Autodesk Fusion 360 part; units mm, degrees
(part 2 of 2)
  constraint equal A46 A113
  constraint equal A46 A102
  constraint equal A46 A91
  constraint equal A46 A108
  constraint equal A46 A95
  constraint equal A46 A130
  constraint equal A142 A148
  constraint equal A148 A166
  constraint equal A148 A164
  constraint equal A148 A174
  constraint equal A148 A172
  constraint equal A148 A158
  constraint equal A148 A156
  constraint coincident L101 L185.end
  measures "d19" distance of L0.end L6.end
  measures "d20" distance of L8.end L11.end
  measures "d51" distance of L0.end L8.end
  measures "d144" distance of L78.start L78.end
  measures "d168" distance of L114.end L115.end
  measures "d179" distance of L159.start L159.end
  measures "d275" diameter of A69
  measures "d276" diameter of A149
  measures "d277" diameter of A179
  measures "d279" diameter of A246
  measures "d280" diameter of A185
  measures "d281" diameter of A187
  measures "d282" diameter of A46
  measures "d283" diameter of A148
extrude "Extrude4" cut sketch "Sketch2" against normal blind 3 contours A46 | A53 | A57 | A58 | A59 | A62 | A63 | A64 | A67 | A68 | A69 | A72 | A73 | A74 | A76 | A77 | A78 | A82 | A83 | A84 | A89 | A91 | A93 | A95 | A97 A120 A139 | A99 | A102 | A104 | A105 | A108 | A111 | A112 | A113 | A116 | A117 | A121 | A124 | A125 | A126 | A129 | A130 | A131 | A134 | A135 | A136 | A141 | A142 | A145 | A147 | A148 | A149 | A155 | A156 | A157 | A158 | A159 | A163 | A164 | A165 | A166 | A167 | A171 | A172 | A173 | A174 | A175 | A201 | A202 | A206 | A207 | A208 | A209 | A210 | A214 | A215 | A216 | A217 | A218 | A219 | A220 | A224 | A225 | A226 | A227 | A228 | A229 | A230 | A234 | A235 | A236 | A237 | A238 | A239 | A240 | A241 | A242 | A243 | A244 | A245 | A246 | A253 | A254 | A255 | A258 | A259 | A260 | A263 | A264 | A265 | A268 | A269 | A270 | A273 | A274 | A275 | A280 | A281 bodies 1
extrude "Extrude5" add sketch "Sketch2" along normal blind 3 separate body contours L0 L5 L34 L35 L36 L37 L107 | L0 L35 L81 L104 L105 L106 L107 | L5 L12 L13 L51 L81 L107 L109 L227 | L0 L7 L81 L100 L101 L102 L103 | L0 L1 L6 L7 L8 L9 L103 | L12 L79 L81 L106 A262 A271 | L10 L79 L81 L102 A261 A267 | L81 L223 A261 L224 A262 | L12 L79 L80 L94 A272 | L1 L10 L11 L48 L81 L103 L108 L226 | L79 L223 A262 | L12 A271 L227 A272 L228 | L79 A272 L228 | L79 L93 L94 L95 A257 | L86 A123 L153 L156 L157 L158 | L10 L225 A266 A267 L226 | L79 L225 A267 | L95 L221 A257 | L93 L221 A256 L222 A257 | L86 A127 L152 L153 | L10 L78 L79 L90 A266 | A75 L93 L95 A256 | L79 L89 L90 L91 A252 | A75 L70 L71 A79 L93 | L146 A127 L147 A128 L152 | A127 L147 L152 | L92 L144 A122 L145 A123 | L89 L219 A252 | L91 L219 A251 L220 A252 | L83 A101 L155 L160 L161 L162 | A79 A80 L93 L95 | L88 L92 L96 L97 L98 L99 L110 L111 L112 L119 L121 L122 L123 L134 A101 A103 A114 A115 L141 A122 A132 L149 A133 L161 | A55 L89 L91 A251 | L83 A109 L154 L155 | A80 L72 A81 L73 L93 | L98 L99 L148 A132 L149 A133 | L62 A55 L63 A56 L91 | A81 L93 L95 L148 | A56 A60 L89 L91 | L138 A109 A110 L139 | L97 L98 L140 A114 A115 L141 | L88 L134 A101 A103 | L64 A60 L65 A61 L91 | A61 L89 L91 L140 | A43 A44 A45 L54 L55 L58 A50 L59 A51 L124 A85 L125 A86 | L56 L57 A47 A48 A49 A52 L60 A54 L61 L126 A87 L127 A88 L132 A98 L133 A100 L136 A106 L137 A107 | L66 A65 L67 A66 A196 L186 A197 L187 | L68 A70 L69 A71 | L128 A90 L129 A92 L164 A143 L165 A144 | L130 A94 L131 A96 L142 A118 L143 A119 L150 A137 L151 A138 | L163 A140 L166 A146 L167 L168 A150 | L173 A160 L174 A161 L175 L176 A162 | L169 A152 L170 A153 L171 L172 A154 | L177 A168 L178 A169 L179 L180 A170 | L188 A198 A199 L189 L190 A200 L191 L192 L193 A203 L194 L195 A204 L196 A205 L197 | A211 L198 L199 A212 L200 L201 A213 L202 | A221 L203 L204 A222 L205 L206 A223 L207 | A231 L208 L209 A232 L210 L211 A233 L212 | A241 | A242 | A243 | A244 | A245 | A246 makes body 2 at (38, -54.1667, 5) makes body 3 at (82.525, -52, 5) makes body 4 at (-92.475, -52, 5) makes body 5 at (-92.4738, 28, 5) makes body 6 at (-92.475, -12, 5) makes body 7 at (82.5262, 28, 5) makes body 8 at (82.525, -12, 5) makes body 9 at (-30.9636, -88.4737, 5) makes body 10 at (-32.5743, -39.2034, 8) makes body 11 at (25.9636, -31.5263, 8) makes body 12 at (27.5743, -80.7966, 8) makes body 13 at (-2.389, 50.3871, 5) makes body 14 at (-1.3541, -12.4596, 5) makes body 15 at (28.8882, 18.9183, 5) makes body 16 at (-33.8882, 19.0817, 8)
sketch "Sketch5" plane through (0, 0, 8) normal (0, 0, 1) x (-1, 0, 0)
  circle A0 centre (90.029, 26.5184) radius 1.425
  circle A1 centre (-45, 12) radius 1.425
  circle A2 centre (86, 66.5) radius 1.175
  circle A3 centre (-45, -32) radius 1.175
  circle A4 centre (50, -32) radius 1.175
  circle A5 centre (90, 66.5) radius 1.425
  circle A6 centre (-89, 26.5) radius 1.175
  circle A7 centre (-45.0037, -28) radius 1.425
  line L0 (-42, 23.5) -> (47, 23.5)
  line L1 (47, 23.5) -> (47, 15.996)
  line L2 (47, 15.996) -> (47.0104, 8.2491)
  arc A8 (47.0104, 8.2491) -> (47, 7.9983) centre (50, 8) ccw
  line L3 (47, 7.9983) -> (47, -24.0028)
  line L4 (47, -24.0028) -> (47.0072, -31.7917)
  arc A9 (47.0072, -31.7917) -> (47, -31.9983) centre (50, -32) ccw
  line L5 (47, -31.9983) -> (47, -61.5)
  line L6 (47, -61.5) -> (38.5028, -61.5)
  line L7 (-42, -61.5) -> (-42, 23.5)
  circle A10 centre (54, 26.5) radius 1.175
  circle A11 centre (49.9963, -28) radius 1.425
  circle A12 centre (-45, 8) radius 1.175
  circle A13 centre (-45, 16) radius 1.175
  circle A14 centre (-85, 66.5) radius 1.425
  circle A15 centre (-45, -24) radius 1.175
  circle A16 centre (50, -24) radius 1.175
  circle A17 centre (50, 16) radius 1.175
  circle A18 centre (50, 12) radius 1.425
  circle A19 centre (-81, 66.5) radius 1.175
  circle A20 centre (86.029, 26.5184) radius 1.175
  circle A21 centre (50, 26.5) radius 1.425
  circle A22 centre (50, 8) radius 1.175
  circle A23 centre (46, 26.5) radius 1.175
  circle A24 centre (-45, 26.5) radius 1.425
  circle A25 centre (-81, 26.5) radius 1.175
  circle A26 centre (94.029, 26.5184) radius 1.175
  circle A27 centre (-49, 26.5) radius 1.175
  circle A28 centre (-41, 26.5) radius 1.175
  circle A29 centre (-85, 26.5) radius 1.425
  circle A30 centre (-89, 66.5) radius 1.175
  circle A31 centre (94, 66.5) radius 1.175
  line L8 (-92.5, -40.1151) -> (-89.5, -40.1151)
  line L9 (-89.5, -40.1151) -> (-89.5, 23.542)
  arc A32 (-89.5, 23.542) -> (-88.996, 23.5) centre (-89, 26.5) ccw
  line L10 (-88.996, 23.5) -> (-81.2491, 23.5104)
  arc A33 (-81.2491, 23.5104) -> (-81.0018, 23.5) centre (-81, 26.5) ccw
  line L11 (-81.0018, 23.5) -> (-48, 23.5)
  line L12 (-48, 23.5) -> (-48, 15.996)
  line L13 (-48, 15.996) -> (-47.9896, 8.2491)
  arc A34 (-47.9896, 8.2491) -> (-48, 7.9983) centre (-45, 8) ccw
  line L14 (-48, 7.9983) -> (-48, -24.0028)
  line L15 (-48, -24.0028) -> (-47.9928, -31.7917)
  arc A35 (-47.9928, -31.7917) -> (-48, -32.0017) centre (-45, -32) ccw
  line L16 (-48, -32.0017) -> (-48, -61.5)
  line L17 (-48, -61.5) -> (-59, -61.5)
  line L18 (-59, -61.5) -> (-59, -67.5)
  line L19 (-59, -67.5) -> (-67.5, -67.5)
  line L20 (-67.5, -67.5) -> (-67.5, -70.5)
  line L21 (-67.5, -70.5) -> (-17.5, -70.5)
  line L22 (-17.5, -70.5) -> (-17.5, -97.5)
  line L23 (-17.5, -97.5) -> (-67.5, -97.5)
  line L24 (-67.5, -97.5) -> (-67.5, -102.5)
  line L25 (-67.5, -102.5) -> (-12.5, -102.5)
  line L26 (-12.5, -102.5) -> (-12.5, -67.5)
  line L27 (-12.5, -67.5) -> (17.5, -67.5)
  line L28 (17.5, -67.5) -> (17.5, -102.5)
  line L29 (17.5, -102.5) -> (72.5, -102.5)
  line L30 (72.5, -102.5) -> (72.5, -97.5)
  line L31 (72.5, -97.5) -> (22.5, -97.5)
  line L32 (22.5, -97.5) -> (22.5, -70.5)
  line L33 (22.5, -70.5) -> (72.5, -70.5)
  line L34 (72.5, -70.5) -> (72.5, -67.5)
  line L35 (72.5, -67.5) -> (64, -67.5)
  line L36 (64, -67.5) -> (64, -61.5)
  line L37 (64, -61.5) -> (53, -61.5)
  line L38 (53, -61.5) -> (53, 23.5)
  line L39 (53, 23.5) -> (94.5, 23.5)
  line L40 (94.5, 23.5) -> (94.5, -40.1151)
  line L41 (94.5, -40.1151) -> (97.5, -40.1151)
  line L42 (97.5, -40.1151) -> (97.5, 69.5047)
  line L43 (97.5, 69.5047) -> (86.2491, 69.4896)
  arc A36 (86.2491, 69.4896) -> (86, 63.5) centre (86, 66.5) ccw
  line L44 (86, 63.5) -> (94, 63.5)
  line L45 (94, 63.5) -> (94.5, 63.5)
  line L46 (94.5, 63.5) -> (94.5, 29.4812)
  arc A37 (94.5, 29.4812) -> (94.361, 29.5) centre (94.029, 26.5184) ccw
  line L47 (94.361, 29.5) -> (59, 29.5)
  line L48 (59, 29.5) -> (47, 41.5)
  line L49 (47, 41.5) -> (47, 91.5)
  line L50 (47, 91.5) -> (41, 91.5)
  line L51 (41, 91.5) -> (41, 29.5)
  line L52 (41, 29.5) -> (-36, 29.5)
  line L53 (-36, 29.5) -> (-36, 91.5)
  line L54 (-36, 91.5) -> (-42, 91.5)
  line L55 (-42, 91.5) -> (-42, 41.5)
  line L56 (-42, 41.5) -> (-54, 29.5)
  line L57 (-54, 29.5) -> (-89, 29.5)
  arc A38 (-89, 29.5) -> (-89.5, 29.458) centre (-89, 26.5) ccw
  line L58 (-89.5, 29.458) -> (-89.5, 63.5)
  line L59 (-89.5, 63.5) -> (-89, 63.5)
  line L60 (-89, 63.5) -> (-81, 63.5)
  arc A39 (-81, 63.5) -> (-81.004, 69.5) centre (-81, 66.5) ccw
  line L61 (-81.004, 69.5) -> (-88.7509, 69.4896)
  arc A40 (-88.7509, 69.4896) -> (-89.2523, 69.4894) centre (-89, 66.5) ccw
  line L62 (-89.2523, 69.4894) -> (-92.5, 69.4894)
  line L63 (-92.5, 69.4894) -> (-92.5, -40.1151)
  circle A41 centre (-57.5, -100) radius 1.15
  circle A42 centre (-57.5, -100) radius 1.15
  circle A43 centre (-42.5, -100) radius 1.15
  circle A44 centre (-27.5, -100) radius 1.15
  circle A45 centre (32.5, -100) radius 1.15
  circle A46 centre (47.5, -100) radius 1.15
  circle A47 centre (62.5, -100) radius 1.15
  circle A48 centre (50, -44) radius 1.175
  circle A49 centre (50, -52) radius 1.175
  circle A50 centre (50, -48) radius 1.425
  circle A51 centre (-45, -52) radius 1.175
  circle A52 centre (-45, -48) radius 1.425
  circle A53 centre (-45, -44) radius 1.175
  circle A54 centre (6.5, -64.5) radius 1.175
  circle A55 centre (-1.5, -64.5) radius 1.175
  circle A56 centre (2.5, -64.5) radius 1.425
  circle A57 centre (-37.5, -64.5) radius 1.425
  circle A58 centre (-33.5, -64.5) radius 1.175
  circle A59 centre (-41.5, -64.5) radius 1.175
  circle A60 centre (42.5, -64.5) radius 1.425
  circle A61 centre (38.5, -64.5) radius 1.175
  circle A62 centre (46.5, -64.5) radius 1.175
  line L64 (-41.4972, -61.5) -> (-42, -61.5)
  line L65 (38.5028, -61.5) -> (-1.4972, -61.5)
  line L66 (-1.4972, -61.5) -> (-41.4972, -61.5)
extrude "Extrude7" cut sketch "Sketch2" against normal blind 5 contours A176 | A177 | A178 | A179 | A180 | A181 | A182 | A183 | A184 | A185 | A186 | A187 | A188 | A189 | A190 | A191 | A192 | A193 | A194 | A195 | A247 | A248 | A249 | A250 bodies 1
extrude "Extrude9" cut sketch "Sketch5" against normal blind 3 contours A41 A42 | A43 | A44 | A45 | A46 | A47 bodies 2
chamfer "Chamfer1" distance 0.5 angle 45 11 edges at (-72.5, 73.5, 0) (-72.5, 102.5, 4) (-72.5, 101.6213, 0.8787) (-87.5, 47.5, 0) (-102.5, -25, 0) (-2.5, -97.5, 0) (97.5, -25, 0) (82.5, 47.5, 0) (67.5, 73.5, 0) (67.5, 102.5, 4) (67.5, 101.6213, 0.8787) on bodies 1
equation "M3_thread = 2.85 mm"
equation "M3_clearance = 3.2 mm"
equation "M2_5_thread = 2.35 mm"
equation "M2_5_clearance = 2.7 mm"
equation "d247 = M2_5_clearance"
equation "d248 = M2_5_clearance"
equation "d249 = M2_5_clearance"
equation "d250 = M2_5_clearance"
equation "d251 = M2_5_clearance"
equation "d252 = M2_5_clearance"
equation "d253 = M2_5_clearance"
equation "d254 = M2_5_clearance"
equation "d256 = M2_5_clearance"
equation "d257 = M2_5_clearance"
equation "d258 = M3_clearance + 1 mm"
equation "d259 = M3_clearance + 1 mm"
equation "d260 = M3_clearance + 1 mm"
equation "d261 = M3_clearance + 1 mm"
equation "d263 = M3_clearance / 2"
equation "d264 = IR_sensor_hole / 2"
equation "d265 = IR_sensor_hole / 2"
equation "d266 = IR_sensor_hole / 2"
equation "IR_sensor_hole = 5 mm"
equation "d268 = IR_sensor_hole / 2"
equation "d269 = IR_sensor_hole / 2"
equation "d270 = IR_sensor_hole / 2"
equation "d271 = IR_sensor_hole / 2"
equation "d272 = IR_sensor_hole / 2"
equation "d273 = IR_sensor_hole / 2"
equation "d274 = IR_sensor_hole / 2"
equation "d275 = M2_5_thread"
equation "d276 = M2_5_thread"
equation "d277 = M2_5_clearance"
equation "d279 = M2_5_thread"
equation "d280 = M3_clearance"
equation "d281 = M3_clearance"
equation "d282 = M3_thread"
equation "d283 = M3_thread"
